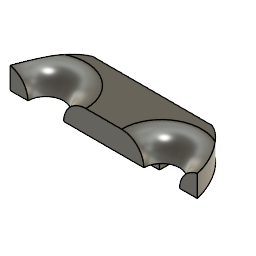
Slopes_v4 (Autodesk Fusion 360 design; units mm, degrees)
Autodesk Fusion 360 part; units mm, degrees
sketch "Sketch1" plane through (0, 0, 0) normal (0, 0, 1) x (1, 0, 0)
  line L0 (0, 0) -> (0, 4) construction
  line L1 (3.7, 2.55) -> (-3.7, 2.55)
  line L2 (-3.7, 2.55) -> (-3.7, 5.45)
  line L3 (-3.7, 5.45) -> (3.7, 5.45)
  line L4 (3.7, 5.45) -> (3.7, 2.55)
  line L5 (3.7, 2.55) -> (-3.7, 5.45) construction
  line L6 (-3.7, 2.55) -> (3.7, 5.45) construction
  line L7 (-6.5, 0) -> (6.5, 0)
  circle A0 centre (6.5, 0) radius 2
  circle A1 centre (-6.5, 0) radius 2
  line L8 (-6.7, 5.45) -> (6.7, 5.45)
  line L9 (-4.5, 0) -> (4.5, 0)
  line L10 (-6.5, 0) -> (-10.5, 0)
  line L11 (6.5, 0) -> (10.5, 0)
  spline S0 degree 5 poles (-6.7, 5.45) (-6.8999, 5.3655) (-7.2917, 5.1615) (-7.8549, 4.7505) (-8.5591, 4.0183) (-9.3533, 2.8757) (-9.896, 1.8161) (-10.2304, 0.9413) (-10.4163, 0.3201) (-10.5, 0) knots 0 0 0 0 0 0 0.2 0.4 0.6 0.8 1 1 1 1 1 1
  line L12 (-6.1899, 5.6656) -> (-7.2101, 5.2344)
  spline S1 degree 5 poles (6.7, 5.45) (6.8999, 5.3655) (7.2917, 5.1615) (7.8549, 4.7505) (8.5591, 4.0183) (9.3533, 2.8757) (9.896, 1.8161) (10.2304, 0.9413) (10.4163, 0.3201) (10.5, 0) knots 0 0 0 0 0 0 0.2 0.4 0.6 0.8 1 1 1 1 1 1
  line L13 (-10.2769, 0.8531) -> (-10.7231, -0.8531)
  line L14 (6.1899, 5.6656) -> (7.2101, 5.2344)
  line L15 (10.2769, 0.8531) -> (10.7231, -0.8531)
  point P0 (0, 4)
  dimension "d1" = 4
  dimension "d2" = 7.4
  dimension "d3" = 2.9
  dimension "d4" = 13
  dimension "d5" = 4
  dimension "d6" = 4
  dimension "d8" = 3
  dimension "d9" = 4
  dimension "d10" = 4
  dimension "d11" = 3
  constraint coincident L0.start origin
  constraint vertical L0
  constraint horizontal L1
  constraint perpendicular L1 L2
  constraint parallel L1 L3
  constraint parallel L2 L4
  constraint coincident L5 P0
  constraint coincident L6 P0
  constraint coincident P0 L0.end
  constraint midpoint L0.start L7
  constraint perpendicular L0 L7
  constraint coincident L7.end A0.centre
  constraint coincident L7.start A1.centre
  constraint coincident A1 L9.start
  constraint coincident L7 L9.start
  constraint coincident A0 L9.end
  constraint coincident L7 L9.end
  constraint parallel L7 L10
  constraint parallel L7 L11
  constraint collinear L3 L8
  constraint midpoint L8.start L12
  constraint midpoint L10.end L13
  constraint symmetric L0 L8.start L8.end
  constraint symmetric L0 L10.end L11.end
  constraint symmetric L0 L12.start L14.start
  constraint symmetric L0 L12.end L14.end
  constraint symmetric L0 L13.start L15.start
  constraint symmetric L0 L13.end L15.end
  measures "d1" distance of L0.start P0
  measures "d2" distance of L2.end L3.end
  measures "d3" distance of L1.end L2.end
  measures "d4" distance of L7.start L7.end
  measures "d5" diameter of A0
  measures "d6" diameter of A1
  measures "d8" distance of L2 L8.start
  measures "d9" distance of L7.start L10.end
  measures "d10" distance of L7.end L11.end
  measures "d11" distance of L4 L8.end
extrude "Extrude1" add sketch "Sketch1" along normal blind 2.5 contours L1 L2 L4 L7 A0 A1 L8 L9 L10 L11 S0 S1 | L1 L2 L3 L4 L8
fillet "Fillet1" radius 2.5 1 edges at (-6.5, 2, 2.5)
fillet "Fillet2" radius 2.5 1 edges at (6.5, 2, 2.5)
extrude "Extrude2" add sketch "Sketch1" against normal blind 2 contours L1 L2 L3 L4 L8
chamfer "Chamfer1" distance 0.1 distance2 2 4 edges at (0, 2.55, -2) (-3.7, 4, -2) (0, 5.45, -2) (3.7, 4, -2) measured on face at (-1.2333, 3.5167, -2) measured on face at (-1.2333, 3.5167, -2) measured on face at (-1.2333, 3.5167, -2) measured on face at (-1.2333, 3.5167, -2) tangent chain off
